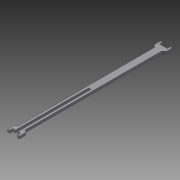
# Autodesk Inventor part: Effector_Arm
Saved by Autodesk Inventor 2014 (Build 180170000, 170)
## iProperties
Created: 2014-08-27
Part Number: Effector_Arm
Material: Generic
Document SubType Name: Modeling
Designer: ThatOtherGuy
Density: 1 g/cm^3
Appearance: Default
Author: ThatOtherGuy
Autodesk Inventor part; units mm, degrees
ref_plane "YZ Plane" through (0, 0, 0) normal (1, 0, 0) x (0, 1, 0)
ref_plane "XZ Plane" through (0, 0, 0) normal (0, 1, 0) x (-1, 0, 0)
ref_plane "XY Plane" through (0, 0, 0) normal (0, 0, 1) x (1, 0, 0)
sketch "Sketch1" plane through (0, 0, 0) normal (0, 0, 1) x (1, 0, 0)
  line L0 (15, 0) -> (12.5, 0)
  line L1 (12.5, 0) -> (12.5, 4)
  line L2 (2.5, 4) -> (2.5, 0)
  line L3 (2.5, 0) -> (0, 0)
  line L4 (12.5, 4) -> (9.0875, 4)
  line L5 (9.0875, 4) -> (9.0875, 97)
  line L6 (9.0875, 97) -> (5.9125, 97)
  line L7 (5.9125, 97) -> (5.9125, 4)
  line L8 (5.9125, 4) -> (2.5, 4)
  line L9 (0, 194) -> (2.5, 194)
  line L10 (2.5, 194) -> (2.5, 190)
  line L11 (2.5, 190) -> (12.5, 190)
  line L12 (12.5, 190) -> (12.5, 194)
  line L13 (12.5, 194) -> (15, 194)
  line L14 (0, 194) -> (0, 188)
  line L15 (0, 188) -> (3.25, 184.75)
  line L16 (3.25, 184.75) -> (3.25, 9.25)
  line L17 (0, 0) -> (0, 6)
  line L18 (0, 6) -> (3.25, 9.25)
  line L19 (15, 0) -> (15, 6)
  line L20 (15, 6) -> (11.75, 9.25)
  line L21 (11.75, 9.25) -> (11.75, 184.75)
  line L22 (11.75, 184.75) -> (15, 188)
  line L23 (15, 188) -> (15, 194)
  dimension "d1" = 10
  dimension "d2" = 3.175
  dimension "d4" = 194
  dimension "d7" = 97
  dimension "d10" = 6
  dimension "d13" = 15
  dimension "d14" = 45
  dimension "d15" = 4
  dimension "d16" = 8.5
  constraints: 48 end point, 12 equal length, 10 parallel, 7 perpendicular, 4 collinear, 2 horizontal alignment, 1 horizontal
  measures "d1" distance between parallel lines of L2 L1
  measures "d2" distance of L5.end L6.end
  measures "d4" distance of L3.end L9.start
  measures "d7" distance between parallel lines of L3 L6
  measures "d10" distance of L3.end L17.end
  measures "d13" distance of L3.end L0.start
  measures "d14" angle of L16 L18
  measures "d15" distance between parallel lines of L3 L8
  measures "d16" distance between parallel lines of L21 L16
extrude "Extrusion1" add sketch "Sketch1" along normal blind 3.175
equation "\"d2\" = THICKA"
equation "\"d7\" = 0.5 * d4"
equation "\"d8\" = THICKA"
equation "\"THICKA\" = 3.175"
equation "\"THICKB\" = 6.731"
equation "\"THICKC\" = 12.7"
body "Solid1"
